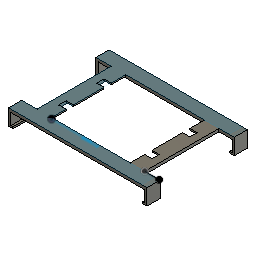
PiSheet backpack (Autodesk Fusion 360 design; units mm, degrees)
part number: 2026-08-13-06-21-30-213
Autodesk Fusion 360 part; units mm, degrees
note: some values were not read from the file. Chosen so that the rebuilt part matches the saved one: which face or edge a step refers to.
sketch "スケッチ1" plane through (0, 0, 0) normal (1, 0, 0) x (0, 0, -1)
  line L0 (0, 0) -> (-51, 0)
  line L1 (-51, 0) -> (-51, 9)
  line L2 (-51, 9) -> (0, 9)
  line L3 (0, 9) -> (0, 0)
  line L4 (-51, 9) -> (-60, 9)
  line L5 (-60, 9) -> (-60, 0)
  line L6 (-60, 0) -> (-51, 0)
  line L7 (-51, 0) -> (-51, 9)
  line L8 (0, 9) -> (9, 9)
  line L9 (9, 9) -> (9, 0)
  line L10 (9, 0) -> (0, 0)
  line L11 (0, 0) -> (0, 9)
  dimension "d1" = 51
  dimension "d2" = 9
  dimension "d3" = 9
  constraint horizontal L0
  constraint vertical L1
  constraint horizontal L2
  constraint vertical L3
  constraint coincident L0.start L3.end
  constraint horizontal L4
  constraint vertical L5
  constraint horizontal L6
  constraint vertical L7
  constraint horizontal L8
  constraint vertical L9
  constraint horizontal L10
  constraint vertical L11
  measures "d1" distance of L0.start L0.end
  measures "d2" distance of L0.start L2.end
  measures "d3" distance of L1.end L4.end
extrude "押し出し1" add sketch "スケッチ1" along normal blind 1 contours L3 L8 L9 L10 L11 | L1 L4 L5 L6 L7 makes body 1 at (0, 6, 57) makes body 2 at (0, 6, -3)
box "直方体プリミティブ1" add length 1.2 width 9 height 1 placed x (0, 1, 0) y (0, 0, 1) z (1, 0, 0) at (1, 0, 51) bodies 1
box "直方体プリミティブ2" add length 1.2 width 9 height 1 placed x (0, 1, 0) y (0, 0, 1) z (1, 0, 0) at (1, 0, -9) bodies 2
extrude "押し出し2" add 2 faces at (0.3333, 9, 54) (0.3333, 9, -3) along direction (0, 1, 0) blind 2 on bodies 1 2 bodies 1 2
box "直方体プリミティブ3" add length 1 width 9 height 90 placed x (0, -1, 0) y (0, 0, -1) z (1, 0, 0) at (1, 11, 60) bodies 1
box "直方体プリミティブ4" add length 1 width 9 height 90 placed x (0, -1, 0) y (0, 0, -1) z (1, 0, 0) at (1, 11, 0) bodies 2
box "直方体プリミティブ5" add length 51 width 10 height 1 placed x (0, 0, 1) y (1, 0, 0) z (0, 1, 0) at (10, 11, 0) separate body makes body 3
extrude "押し出し3" add 1 faces at (16.6667, 11, 17) along direction (0, -1, 0) blind 1 on bodies 3 bodies 1 3 2
extrude "押し出し4" cut 1 faces at (16.6667, 12, 17) along direction (0, -1, 0) blind 1 on bodies 1 bodies 1
sketch "スケッチ7" plane through (0, 11, 0) normal (0, 1, 0) x (-1, 0, 0)
  line L0 (0, 51) -> (0, 60)
  line L1 (0, 60) -> (-91, 60)
  line L2 (-91, 60) -> (-91, 51)
  line L3 (-91, 51) -> (-20, 51)
  line L4 (-20, 51) -> (-20, 0)
  line L5 (-20, 0) -> (-91, 0)
  line L6 (-91, 0) -> (-91, -9)
  line L7 (-91, -9) -> (0, -9)
  line L8 (0, -9) -> (0, 0)
  line L9 (0, 0) -> (-10, 0)
  line L10 (-10, 0) -> (-10, 51)
  line L11 (-10, 51) -> (0, 51)
box "直方体プリミティブ6" add length 9 width 90 height 1 placed x (0, 0, 1) y (-1, 0, 0) z (0, -1, 0) at (91, 10, 51) bodies 1
box "直方体プリミティブ7" add length 9 width 90 height 1 placed x (0, 0, 1) y (-1, 0, 0) z (0, -1, 0) at (91, 10, -9) bodies 1
extrude "押し出し5" add 1 faces at (91, 10.3333, 57) along direction (1, 0, 0) blind 2 on bodies 1 bodies 1
extrude "押し出し6" add 1 faces at (91, 10.3333, -6) along direction (1, 0, 0) blind 2 on bodies 1 bodies 1
extrude "押し出し7" add 1 faces at (93, 10.3333, -6) along direction (1, 0, 0) blind 1 on bodies 1 bodies 1
extrude "押し出し8" add 1 faces at (93, 10.3333, 57) along direction (1, 0, 0) blind 1 on bodies 1 bodies 1
box "直方体プリミティブ8" add length 9 width 1 height 11 placed x (0, 0, -1) y (1, 0, 0) z (0, -1, 0) at (93, 9, 60) bodies 1
extrude "押し出し9" cut 1 faces at (93.6667, -2, 57) along direction (0, 1, 0) blind 2 on bodies 1 bodies 1
box "直方体プリミティブ9" add length 9 width 1 height 9 placed x (0, 0, -1) y (1, 0, 0) z (0, -1, 0) at (93, 9, 0) bodies 1
box "直方体プリミティブ10" add length 1.2 width 9 height 1 placed x (0, 1, 0) y (0, 0, -1) z (-1, 0, 0) at (93, 0, 0) bodies 1
box "直方体プリミティブ11" add length 1.2 width 9 height 1 placed x (0, 1, 0) y (0, 0, -1) z (-1, 0, 0) at (93, 0, 60) bodies 1
sketch "スケッチ14" plane through (92, 0, 0) normal (-1, 0, 0) x (0, 0, 1)
  line L0 (0, 1.2) -> (-9, 1.2)
  line L1 (-9, 1.2) -> (-9, 0)
  line L2 (-9, 0) -> (0, 0)
  line L3 (0, 0) -> (0, 1.2)
sketch "スケッチ15" plane through (0, 11, 0) normal (0, 1, 0) x (-1, 0, 0)
  line L0 (0, 51) -> (0, 60)
  line L1 (0, 60) -> (-94, 60)
  line L2 (-94, 60) -> (-94, 51)
  line L3 (-94, 51) -> (-20, 51)
  line L4 (-20, 51) -> (-20, 0)
  line L5 (-20, 0) -> (-94, 0)
  line L6 (-94, 0) -> (-94, -9)
  line L7 (-94, -9) -> (0, -9)
  line L8 (0, -9) -> (0, 0)
  line L9 (0, 0) -> (-10, 0)
  line L10 (-10, 0) -> (-10, 51)
  line L11 (-10, 51) -> (0, 51)
  line L12 (-94, 51) -> (-84, 51)
  constraint coincident L2.end L3.start
  constraint coincident L3 L12.end
box "直方体プリミティブ12" add length 51 width 10 height -1 placed x (0, 0, 1) y (1, 0, 0) z (0, 1, 0) at (74, 11, 0) bodies 1
sketch "スケッチ17" plane through (0, 11, 0) normal (0, 1, 0) x (-1, 0, 0)
  line L0 (-84, 0) -> (-94, 0)
  line L1 (-94, 0) -> (-94, -9)
  line L2 (-94, -9) -> (0, -9)
  line L3 (0, -9) -> (0, 0)
  line L4 (0, 0) -> (-10, 0)
  line L5 (-10, 0) -> (-10, 51)
  line L6 (-10, 51) -> (0, 51)
  line L7 (0, 51) -> (0, 60)
  line L8 (0, 60) -> (-94, 60)
  line L9 (-94, 60) -> (-94, 51)
  line L10 (-94, 51) -> (-84, 51)
  line L11 (-84, 51) -> (-84, 0)
  line L12 (-74, 0) -> (-74, 51)
  line L13 (-74, 51) -> (-20, 51)
  line L14 (-20, 51) -> (-20, 0)
  line L15 (-20, 0) -> (-74, 0)
  line L16 (-74, 51) -> (-74, 41)
  line L17 (-74, 0) -> (-74, 10)
  line L18 (-74, 41) -> (-79, 41)
  line L19 (-79, 41) -> (-79, 36)
  line L20 (-79, 36) -> (-74, 36)
  line L21 (-74, 36) -> (-74, 41)
  line L22 (-74, 10) -> (-79, 10)
  line L23 (-79, 10) -> (-79, 15)
  line L24 (-79, 15) -> (-74, 15)
  line L25 (-74, 15) -> (-74, 10)
  line L26 (-20, 41) -> (-15, 41)
  line L27 (-15, 41) -> (-15, 36)
  line L28 (-15, 36) -> (-20, 36)
  line L29 (-20, 36) -> (-20, 41)
  line L30 (-20, 15) -> (-15, 15)
  line L31 (-15, 15) -> (-15, 10)
  line L32 (-15, 10) -> (-20, 10)
  line L33 (-20, 10) -> (-20, 15)
  constraint coincident L12.end L13.start
  constraint coincident L12 L16.end
  constraint coincident L12.start L15.end
  constraint coincident L12 L17.end
  constraint horizontal L18
  constraint vertical L19
  constraint horizontal L20
  constraint vertical L21
  constraint horizontal L22
  constraint vertical L23
  constraint horizontal L24
  constraint vertical L25
  constraint horizontal L26
  constraint vertical L27
  constraint horizontal L28
  constraint vertical L29
  constraint coincident L14 L26.start
  constraint horizontal L30
  constraint vertical L31
  constraint horizontal L32
  constraint vertical L33
  constraint coincident L14 L30.start
extrude "押し出し10" cut sketch "スケッチ17" against normal blind 10 contours L12 L22 L23 L24 L25 | L14 L30 L31 L32 L33 | L12 L18 L19 L20 L21 | L14 L26 L27 L28 L29 bodies 1
sketch "スケッチ18" plane through (0, 11, 0) normal (0, 1, 0) x (-1, 0, 0)
  line L0 (-20, 51, -1) -> (-47, 51, -1)
  line L1 (-47, 51, -1) -> (-42, 51, -1)
  line L2 (-42, 51, -1) -> (-52, 51, -1)
  line L3 (-52, 51, -1) -> (-52, 52, -1)
  line L4 (-52, 52, -1) -> (-42, 52, -1)
  line L5 (-42, 52, -1) -> (-42, 51, -1)
  point P0 (-20, 51)
  dimension "d89" = 27
box "直方体プリミティブ13" cut length 1 width 10 height -5 placed x (0, -1, 0) y (-1, 0, 0) z (0, 0, -1) at (52, 10, 51) bodies 1
extrude "押し出し11" add 1 faces at (0, 3.6667, -6) along direction (-1, 0, 0) blind 0.5 on bodies 1 bodies 1
extrude "押し出し12" add 1 faces at (0, 7.3333, 57) along direction (-1, 0, 0) blind 0.5 on bodies 1 bodies 1
extrude "押し出し13" add 2 faces at (94, 10.3333, 57) (94, 6, 54) along direction (1, 0, 0) blind 0.5 on bodies 1 bodies 1
extrude "押し出し14" add 2 faces at (94, 10.3333, -6) (94, 6, -6) along direction (1, 0, 0) blind 0.5 on bodies 1 bodies 1
extrude "押し出し15" add 1 faces at (2, 0.4, 57) along direction (1, 0, 0) blind 0.5 on bodies 1 bodies 1
extrude "押し出し16" add 1 faces at (2, 0.4, -3) along direction (1, 0, 0) blind 0.5 on bodies 1 bodies 1
extrude "押し出し17" add sketch "スケッチ14" along normal blind 0.5 bodies 1
extrude "押し出し18" add 1 faces at (92, 0.4, 54) along direction (-1, 0, 0) blind 0.5 on bodies 1 bodies 1
box "直方体プリミティブ14" add length 50 width 5 height 1 placed x (0, 0, -1) y (1, 0, 0) z (0, -1, 0) at (79, 10, 51) bodies 1
extrude "押し出し19" add 1 faces at (80.6667, 9.6667, 1) along direction (0, 0, -1) blind 1 on bodies 1 bodies 1
box "直方体プリミティブ15" add length 51 width 5 height 1 placed x (0, 0, -1) y (1, 0, 0) z (0, -1, 0) at (10, 10, 51) bodies 1
